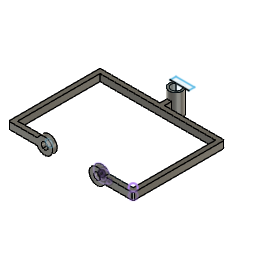
Attache_raspberry (Autodesk Fusion 360 design; units mm, degrees)
Autodesk Fusion 360 part; units mm, degrees
note: some values were not read from the file. Set by a fixed rule: which sketch regions a step uses.
sketch "Esquisse1" plane through (0, 0, 0) normal (0, 0, 1) x (1, 0, 0)
  circle A0 centre (0, 0) radius 2.1
  circle A1 centre (0, 0) radius 3
  dimension "d1" = 4.2
  dimension "d2" = 6
  constraint coincident A0.centre A1.centre
  constraint concentric A0 A1
  measures "d1" diameter of A0
  measures "d2" diameter of A1
extrude "Extrusion1" add sketch "Esquisse1" along normal blind 10 makes body 1
ref_plane "Plan de construction1" through (0, 0, 5) normal (0, 0, 1) x (1, 0, 0)
sketch "Esquisse2" plane through (0, 0, 5) normal (0, 0, 1) x (1, 0, 0)
  line L0 (-1, 0) -> (1, 0)
  line L1 (1, 0) -> (1, -8)
  line L2 (1, -8) -> (-1, -8)
  line L3 (-1, -8) -> (-1, 0)
  line L4 (-27.25, -6) -> (27.25, -6)
  line L5 (27.25, -6) -> (27.25, -8)
  line L6 (27.25, -8) -> (-27.25, -8)
  line L7 (-27.25, -8) -> (-27.25, -6)
  circle A0 centre (0, 0) radius 2
  circle A1 centre (0, 0) radius 3
  line L8 (-27.25, -6) -> (-25.25, -6)
  line L9 (-25.25, -6) -> (-25.25, -46)
  line L10 (-25.25, -46) -> (-27.25, -46)
  line L11 (-27.25, -46) -> (-27.25, -6)
  line L12 (27.25, -6) -> (25.25, -6)
  line L13 (25.25, -6) -> (25.25, -46)
  line L14 (25.25, -46) -> (27.25, -46)
  line L15 (27.25, -46) -> (27.25, -6)
  line L16 (-27.25, -44) -> (-12.25, -44)
  line L17 (-12.25, -44) -> (-12.25, -46)
  line L18 (-12.25, -46) -> (-27.25, -46)
  line L19 (-27.25, -46) -> (-27.25, -44)
  line L20 (0, -23) -> (0, -29)
  line L21 (27.25, -44) -> (12.25, -44)
  line L22 (12.25, -46) -> (27.25, -46)
  line L23 (12.25, -44) -> (12.25, -46)
  dimension "d6" = 54.5
  dimension "d7" = 27.25
  dimension "d8" = 2
  dimension "d9" = 8
  dimension "d10" = 8
  dimension "d11" = 1
  dimension "d12" = 1
  dimension "d13" = 2
  dimension "d14" = 2
  dimension "d15" = 40
  dimension "d16" = 40
  dimension "d17" = 2
  dimension "d18" = 15
  dimension "d52" = 50.5
  constraint horizontal L0
  constraint vertical L1
  constraint horizontal L2
  constraint vertical L3
  constraint horizontal L4
  constraint vertical L5
  constraint horizontal L6
  constraint vertical L7
  constraint coincident L2 L5.end
  constraint coincident A0.centre A1.centre
  constraint concentric A0 A1
  constraint horizontal L8
  constraint vertical L9
  constraint horizontal L10
  constraint vertical L11
  constraint horizontal L12
  constraint vertical L13
  constraint horizontal L14
  constraint vertical L15
  constraint horizontal L16
  constraint vertical L17
  constraint horizontal L18
  constraint vertical L19
  constraint coincident L11 L16.start
  constraint coincident L9.end L18
  constraint perpendicular L4 L20
  constraint symmetric L16.start L20 L21.start
  constraint symmetric L16.end L20 L21.end
  constraint symmetric L17.end L20 L22.start
  constraint symmetric L10.end L20 L14.end
  measures "d6" distance of L5.end L6.end
  measures "d7" distance of A0.centre L7
  measures "d8" distance of L4.start L6.end
  measures "d9" distance of A0.centre L2
  measures "d10" distance of L0 L2
  measures "d11" distance of L3 A0.centre
  measures "d12" distance of L1 A0.centre
  measures "d13" distance of L4.end L12.end
  measures "d14" distance of L4.start L8.end
  measures "d15" distance of L4.end L14.end
  measures "d16" distance of L4.start L10.end
  measures "d17" distance of L16.end L17.end
  measures "d18" distance of L16.start L16.end
  measures "d52" distance of L9 L13
extrude "Extrusion2" add sketch "Esquisse2" along normal blind -1.5 and the other way blind -1.5 separate body contours L1 L3 L4 A1 | L1 L2 L3 L4 L6 | L3 L4 L6 L9 | L1 L4 L6 L13 | L4 L6 L7 L8 L9 L11 | L4 L5 L6 L12 L13 L15 | L6 L9 L11 L16 | L6 L13 L15 L21 | L9 L16 L17 L18 | L9 L10 L11 L16 L18 L19 | L13 L14 L15 L21 L22 | L13 L21 L22 L23 makes body 2
sketch "Esquisse3" plane through (0, -44, 0) normal (0, 1, 0) x (-1, 0, 0)
  line L0 (12.25, 6.5) -> (12.25, 3.5)
  line L1 (12.25, 3.5) -> (25.25, 3.5)
  line L2 (25.25, 3.5) -> (25.25, 6.5)
  line L3 (25.25, 6.5) -> (12.25, 6.5)
  circle A0 centre (11.5, 4.9931) radius 3.5
  circle A1 centre (11.5, 4.9931) radius 1.475
  circle A2 centre (-11.5, 5) radius 3.5
  circle A3 centre (-11.5, 5) radius 1.475
  line L4 (-27.25, 3.5) -> (-27.25, 6.5)
  line L5 (27.25, 3.5) -> (27.25, 6.5)
  point P0 (-12.25, 3.5)
  dimension "d23" = 7
  dimension "d25" = 2.95
  dimension "d26" = 7
  dimension "d28" = 2.95
  dimension "d29" = 23
  dimension "d50" = 15.75
  dimension "d51" = 15.75
  constraint concentric A0 A1
  constraint concentric A2 A3
  measures "d23" diameter of A0
  measures "d25" diameter of A1
  measures "d26" diameter of A2
  measures "d28" diameter of A3
  measures "d29" horizontal distance of A0.centre A2.centre
  measures "d50" distance of A2.centre L4
  measures "d51" distance of A0.centre L5
extrude "Extrusion3" add sketch "Esquisse3" along normal blind -2 and the other way blind 0 contours L0 L1 L3 A0 A1 | L0 L1 L3 A0 A1 | L1 L2 L3 A0 | A2 bodies 2
sketch "Esquisse4" plane through (0, -44, 0) normal (0, 1, 0) x (-1, 0, 0)
  line L0 (-14.6623, 6.5) -> (-25.25, 6.5)
  line L1 (-25.25, 6.5) -> (-25.25, 3.5)
  line L2 (-25.25, 3.5) -> (-14.6623, 3.5)
  circle A0 centre (-11.5, 5) radius 1.475
  circle A1 centre (11.5, 5) radius 1.475
  line L3 (-12.25, 3.7299) -> (-12.25, 6.2701)
  arc A2 (-12.25, 3.7299) -> (-12.25, 6.2701) centre (-11.5, 5) ccw
  arc A3 (-14.6623, 3.5) -> (-14.6623, 6.5) centre (-11.5, 5) ccw
  dimension "d32" = 23
  dimension "d33" = 2.95
  dimension "d34" = 2.95
  constraint coincident A0.centre A2.centre
  measures "d32" distance of A0.centre A1.centre
  measures "d33" diameter of A0
  measures "d34" diameter of A1
extrude "Extrusion4" cut sketch "Esquisse4" against normal blind 2 contours A0 L3 A2 | A0 L3 | A1 bodies 2
fillet "Congé1" radius 0.5 2 edges at (27.25, -6, 5) (-27.25, -6, 5) on bodies 2
fillet "Congé2" radius 0.5 2 edges at (-27.25, -46, 5) (27.25, -46, 5) on bodies 2
sketch "Esquisse5" plane through (0, 0, 10) normal (0, 0, 1) x (-1, 0, 0)
  circle A0 centre (0, 0) radius 2.1
  circle A1 centre (0, 0) radius 3
  line L0 (4, -1.5) -> (-4.0846, -1.5)
  line L1 (-4.0846, -1.5) -> (-4.0846, -4.0007)
  line L2 (-4.0846, -4.0007) -> (4, -4.0007)
  line L3 (4, -4.0007) -> (4, -1.5)
  dimension "d41" = 1.5
  constraint horizontal L0
  constraint vertical L1
  constraint horizontal L2
  constraint vertical L3
  measures "d41" distance of A0.centre L0
extrude "Extrusion5" cut sketch "Esquisse5" against normal blind 10 contours A0 L0 | A0 A1 L0 | A1 L0 L1 L2 L3 picked at (-0.4148, -1.5639) picked at (-0.1983, -2.6871) bodies 1
sketch "Esquisse11" plane through (0, 0, 0) normal (0, 0, 1) x (1, 0, 0)
